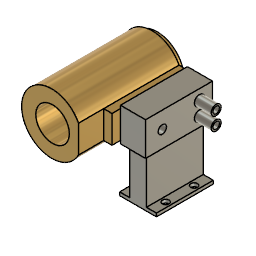
Cylinder (Autodesk Fusion 360 design; units mm, degrees)
Autodesk Fusion 360 part; units mm, degrees
note: some values were not read from the file. Set by a fixed rule: which sketch regions a step uses.
sketch "Main Body Sketch" plane through (0, 0, 0) normal (0, 1, 0) x (1, 0, 0) in component "Cylinder Body"
  circle A0 centre (0, 0) radius 5
  circle A1 centre (0, 0) radius 9
  line L0 (-8, -4.1231) -> (-8, 4.1231)
  dimension "d2" = 10
  dimension "d3" = 4
  dimension "d10" = 8
  constraint coincident A0.centre A1.centre
  constraint coincident A1 L0.start
  constraint coincident A1 L0.end
  constraint vertical L0
  measures "d2" diameter of A0
  measures "d10" distance of A0.centre L0
extrude "Extrude1" add sketch "Main Body Sketch" along normal blind 30 contours A0 | A1 L0 picked at (-7, 0) makes body 1 in component "Cylinder Body"
hole "Hole1" at (-0.25, 0, 0) direction (0, 1, 0) diameter 10 end through all bodies 1 in component "Cylinder Body"
sketch "Oscillating Hole Sketch" plane through (-8, 0, 0) normal (-1, 0, 0) x (0, -1, 0) in component "Cylinder Body"
  line L0 (0, -4.1231) -> (0, 4.1231)
  line L1 (0, 4.1231) -> (-30, 4.1231)
  line L2 (-30, 4.1231) -> (-30, -4.1231)
  line L3 (-30, -4.1231) -> (0, -4.1231)
  line L4 (-15, 4.1231) -> (-15, -4.1231)
  line L5 (0, 0) -> (-30, 0)
  circle A0 centre (-15, 0) radius 1.5
  dimension "d11" = 3
  constraint midpoint L1 L4.start
  constraint midpoint L3 L4.end
  constraint coincident L5.start origin
  constraint midpoint L2 L5.end
  constraint midpoint L5 A0.centre
  measures "d11" diameter of A0
sketch "Intake Hole Sketch" plane through (-8, 0, 0) normal (-1, 0, 0) x (0, -1, 0) in component "Cylinder Body"
  line L0 (0, -4.1231) -> (0, 4.1231)
  line L1 (0, 4.1231) -> (-30, 4.1231)
  line L2 (-30, 4.1231) -> (-30, -4.1231)
  line L3 (-30, -4.1231) -> (0, -4.1231)
  line L4 (-15, 0) -> (-30, 0)
  line L5 (-22.5, 0) -> (-30, 0)
  line L6 (-22.5, 0) -> (-30, 0)
  circle A0 centre (-15, 0) radius 1.25
  point P0 (-26.25, 0)
  dimension "d48" = 2.5
  constraint midpoint L2 L4.end
  constraint midpoint L5 P0
  constraint perpendicular L2 L6
  constraint coincident L4.start A0.centre
  measures "d48" diameter of A0
hole "Hole2" at (-8, 26.25, 0) direction (1, 0, 0) diameter 2 depth 5 tip angle 118 bodies 1 in component "Cylinder Body"
sketch "Sketch5" plane through (0, 30, 0) normal (0, 1, 0) x (-1, 0, 0) in component "Cylinder Body"
  circle A0 centre (0.25, 0) radius 5
  arc A1 (8, 4.1231) -> (8, -4.1231) centre (0, 0) ccw
  line L0 (8, 4.1231) -> (8, -4.1231)
  line L1 (8, -4.1231) -> (8, 4.1231)
  point P0 (8, 4.1231)
  point P1 (8, -4.1231)
  constraint coincident P1 A1.end
sketch "Main Body Sketch (2)" plane through (0, 0, 0) normal (0, 1, 0) x (1, 0, 0) in component "Cylinder Lid"
  circle A0 centre (0, 0) radius 8
  dimension "d26" = 16
  constraint coincident A0.centre origin
  measures "d26" diameter of A0
extrude "Extrude1'" add sketch "Main Body Sketch (2)" along normal blind 1.5 separate body makes body 2 in component "Cylinder Lid"
sketch "Sketch7" plane through (-8, 0, 0) normal (-1, 0, 0) x (0, -1, 0) in component "Cylinder Body"
  circle A0 centre (-26.25, 0) radius 1
  line L0 (0, -4.1231) -> (0, 4.1231)
  line L1 (0, 4.1231) -> (-30, 4.1231)
  line L2 (-30, 4.1231) -> (-30, -4.1231)
  line L3 (-30, -4.1231) -> (0, -4.1231)
  line L4 (-15, 4.1231) -> (-15, -4.1231) construction
  line L5 (-15, 0) -> (0, 0) construction
  line L6 (-7.491, 4.1231) -> (-7.491, -4.1231)
  point P0 (-7.491, 0)
  constraint midpoint L1 L4.start
  constraint midpoint L3 L4.end
  constraint midpoint L4 L5.start
  constraint coincident L5.end origin
  constraint coincident L1 L6.start
  constraint coincident L3 L6.end
  constraint perpendicular L3 L6
  constraint midpoint L6 P0
extrude "Extrude7" add sketch "Sketch7" along normal blind 2.5 contours L1 L2 L3 L6 bodies 1 in component "Cylinder Body"
extrude "Extrude8" cut sketch "Intake Hole Sketch" along normal up to surface (2.5 mm away) contours A0 bodies 1 in component "Cylinder Body"
sketch "Sketch1" plane through (0, 0, 0) normal (1, 0, 0) x (0, 1, 0) in component "Cylinder Mount"
  line L0 (-10, 5) -> (10, 5)
  line L1 (10, 5) -> (10, -5)
  line L2 (10, -5) -> (-10, -5)
  line L3 (-10, -5) -> (-10, 5)
  line L4 (-10, 5) -> (10, -5) construction
  line L5 (10, 5) -> (-10, -5) construction
  line L6 (8.5, -5) -> (-8.4104, -5)
  line L7 (8.5, -5) -> (-8.5, -5)
  line L8 (-8.5, -5) -> (-8.5, -20)
  line L9 (-8.5, -20) -> (8.5, -20)
  line L10 (8.5, -20) -> (8.5, -5)
  dimension "d55" = 20
  dimension "d56" = 10
  dimension "d58" = 1.5
  dimension "d59" = 1.5
  dimension "d60" = 15
  constraint horizontal L0
  constraint perpendicular L0 L1
  constraint parallel L0 L2
  constraint parallel L1 L3
  constraint coincident L4 origin
  constraint coincident L5 origin
  constraint coincident L2 L6.start
  constraint coincident L2 L6.end
  constraint horizontal L7
  constraint vertical L8
  constraint horizontal L9
  constraint vertical L10
  measures "d55" distance of L1.end L2.end
  measures "d56" distance of L0.end L1.end
  measures "d58" distance of L1 L10
  measures "d59" distance of L3 L8
  measures "d60" distance of L7.end L8.end
extrude "Extrude1''" add sketch "Sketch1" along normal mid plane 7.5 separate body contours L0 L1 L2 L3 L6 L7 makes body 3 in component "Cylinder Mount"
extrude "Extrude2" add sketch "Sketch1" along normal mid plane 5 contours L2 L6 L7 L8 L9 L10 bodies 3 in component "Cylinder Mount"
sketch "Sketch2" plane through (-3.75, 0, 0) normal (-1, 0, 0) x (0, -1, 0) in component "Cylinder Mount"
  line L0 (-10, -5) -> (10, -5)
  line L1 (10, -5) -> (10, 5)
  line L2 (10, 5) -> (-10, 5)
  line L3 (-10, 5) -> (-10, -5)
  line L4 (0, 0) -> (10, 0)
  circle A0 centre (-6.25, 0) radius 1
  point P0 (5, 0)
  point P1 (-6.25, 0)
  point P2 (-6.075, 1.9923)
  point P3 (-6.075, -1.9923)
  dimension "d66" = 11.25
  dimension "d75" = 2
  dimension "d76" = 2
  dimension "d77" = 2
  dimension "d82" = 0.175
  dimension "d83" = 0.175
  constraint coincident L4.start origin
  constraint midpoint L1 L4.end
  constraint midpoint L4 P0
  constraint horizontal P0 P1
  constraint coincident P1 A0.centre
  measures "d66" distance of P0 P1
  measures "d75" diameter of A0
  measures "d76" distance of P1 P2
  measures "d77" distance of P1 P3
  measures "d82" horizontal distance of P1 P2
  measures "d83" horizontal distance of P1 P3
hole "Hole1'" at (-3.75, -5, 0) direction (1, 0, 0) diameter 2.5 end through all bodies 3 in component "Cylinder Mount"
hole "Hole3" at (-3.75, 6.075, 1.9923) direction (1, 0, 0) diameter 2 end through all bodies 3 in component "Cylinder Mount"
hole "Hole4" at (-3.75, 6.075, -1.9923) direction (1, 0, 0) diameter 2 end through all bodies 3 in component "Cylinder Mount"
sketch "Sketch3" plane through (2.5, 0, 0) normal (1, 0, 0) x (0, 1, 0) in component "Cylinder Mount"
  circle A0 centre (6.075, -1.9923) radius 1
  circle A1 centre (6.075, 1.9923) radius 1
  circle A2 centre (-5, 0) radius 1.25
  line L0 (-10, -5) -> (10, -5)
  line L1 (10, -5) -> (10, 5)
  line L2 (10, 5) -> (-10, 5)
  line L3 (-10, 5) -> (-10, -5)
  line L4 (8.5, -20) -> (-8.5, -20)
  line L5 (-8.5, -20) -> (-8.5, -19)
  line L6 (-8.5, -19) -> (8.5, -19)
  line L7 (8.5, -19) -> (8.5, -20)
  dimension "d84" = 1
  constraint horizontal L4
  constraint vertical L5
  constraint horizontal L6
  constraint vertical L7
  measures "d84" distance of L4.start L6.end
extrude "Extrude3" add sketch "Sketch3" along normal blind 3 contours L4 L5 L6 L7 bodies 3 in component "Cylinder Mount"
sketch "Sketch4" plane through (0, 0, -19) normal (0, 0, 1) x (-1, 0, 0) in component "Cylinder Mount"
  line L0 (-2.5, -8.5) -> (-2.5, 8.5)
  line L1 (-2.5, 8.5) -> (-5.5, 8.5)
  line L2 (-5.5, 8.5) -> (-5.5, -8.5)
  line L3 (-5.5, -8.5) -> (-2.5, -8.5)
  line L4 (-2.5, 0) -> (-5.5, 0)
  line L5 (-4, 0) -> (-4, 8.5)
  line L6 (-4, 0) -> (-4, -8.5)
  point P0 (-4, 4.25)
  point P1 (-4, -4.25)
  constraint midpoint L0 L4.start
  constraint midpoint L2 L4.end
  constraint midpoint L4 L5.start
  constraint midpoint L1 L5.end
  constraint midpoint L5 P0
  constraint midpoint L3 L6.end
  constraint midpoint L6 P1
hole "Hole5" at (4, 4.25, -19) direction (0, 0, -1) diameter 2 end through all bodies 3 in component "Cylinder Mount"
pattern_linear "R-Pattern1" count 2 spacing 8.5 along (0, -1, 0) of "Hole5" in component "Cylinder Mount"
mirror "Mirror1" about plane through (0, 0, 0) normal (1, 0, 0) of "Extrude3", "Hole5", "R-Pattern1" in component "Cylinder Mount"
sketch "Sketch6" plane through (3.75, 0, 0) normal (1, 0, 0) x (0, 1, 0) in component "Cylinder Mount"
  circle A0 centre (6.075, -1.9923) radius 1
  circle A1 centre (6.075, 1.9923) radius 1
  circle A2 centre (-5, 0) radius 1.25
  line L0 (-10, -5) -> (10, -5)
  line L1 (10, -5) -> (10, 5)
  line L2 (10, 5) -> (-10, 5)
  line L3 (-10, 5) -> (-10, -5)
  circle A3 centre (6.075, 1.9923) radius 1.5
  circle A4 centre (6.075, -1.9923) radius 1.5
  dimension "d121" = 0.5
  dimension "d122" = 0.5
extrude "Extrude4" add sketch "Sketch6" along normal blind 5 contours A3 | A4 bodies 3 in component "Cylinder Mount"
component "Cylinder Body" placed x (-1, 0, 0) y (0, 1, 0) z (0, 0, -1) at (-14.25, -20, 0)
component "Cylinder Lid" placed x (1, 0, 0) y (0, 1, 0) z (0, 0, 1) at (-14.25, 10, 0)
component "Cylinder Mount" placed x (1, 0, 0) y (0, 1, 0) z (0, 0, 1) at (0, 0, 0)
equation "Cylinder_Dia_In = 10 mm"
equation "d2 = Cylinder_Dia_In"
equation "d4 = Cylinder_Length"
equation "Cylinder_Length = 30 mm"
equation "d7 = Cylinder_Dia_In"
equation "d14 = Cylinder_Dia_In / 2"
equation "d61 = ( 7.5 / 2 ) * 1 mm"
equation "d63 = ( 5 / 2 ) * 1 mm"
